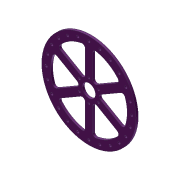
# Autodesk Inventor part: FlyWheelBase
Saved by Autodesk Inventor 2012 (Build 160160000, 160)
## iProperties
Created: 2012-01-20
Part Number: FlyWheelBase
Material: Aluminum-6061
Document SubType Name: Modeling
Designer: JesseK
Mass: 221.849 g
Surface Area: 457.511 cm^2
Volume: 81.8629 cm^3
Density: 2.71 g/cm^3
Author: JesseK
Autodesk Inventor part; units mm, degrees
ref_plane "YZ Plane" through (0, 0, 0) normal (1, 0, 0) x (0, 1, 0)
ref_plane "XZ Plane" through (0, 0, 0) normal (0, 1, 0) x (-1, 0, 0)
ref_plane "XY Plane" through (0, 0, 0) normal (0, 0, 1) x (1, 0, 0)
sketch "Sketch1" plane through (0, 0, 0) normal (0, 0, 1) x (1, 0, 0)
  circle A0 centre (0, 0) radius 101.6
  circle A1 centre (0, 0) radius 14.2875
  dimension "d0" = 203.2
  dimension "d1" = 28.575
  constraints: 2 centre point, 1 coincident
  measures "d0" diameter of A0
  measures "d1" diameter of A1
extrude "Extrusion1" add sketch "Sketch1" along normal blind 4.7625
sketch "Sketch4" plane through (0, 0, 4.7625) normal (0, 0, 1) x (1, 0, 0)
  circle A0 centre (0, 0) radius 101.6 projected
  circle A1 centre (0, 92.075) radius 2.8063
  line L0 (0, 0) -> (0, 101.6) construction
  circle A2 centre (0, 0) radius 92.075 construction
  dimension "d58" = 9.525
  constraints: 2 end point, 2 vertical alignment, 1 centre point, 1 coincident, 1 point on line, 1 vertical, 3 other
extrude "Extrusion5" cut sketch "Sketch4" against normal through all contours A1
pattern_circular "Circular Pattern3" count 24 over 360 about axis through (0, 0, -10) along (0, 0, 1) of "Extrusion5"
sketch "Sketch6" plane through (0, 0, 4.7625) normal (0, 0, 1) x (1, 0, 0)
  circle A0 centre (0, 0) radius 101.6 projected
  circle A1 centre (0, 23.8125) radius 2.3813
  circle A2 centre (0, 0) radius 23.8125 construction
  line L0 (0, 23.8125) -> (0, 0) construction
  dimension "d68" = 47.625
  dimension "d69" = 4.7625
  constraints: 2 end point, 1 centre point, 1 coincident, 1 vertical, 1 vertical alignment, 2 other
  measures "d69" diameter of A1
extrude "Extrusion6" cut sketch "Sketch6" against normal through all contours A1
pattern_circular "Circular Pattern4" count 6 over 360 about axis through (0, 0, -10) along (0, 0, 1) of "Extrusion6"
sketch "Sketch7" plane through (0, 0, 4.7625) normal (0, 0, 1) x (1, 0, 0)
  circle A0 centre (-20.6222, -11.9062) radius 2.3813 projected
  circle A1 centre (-20.6222, 11.9062) radius 2.3813 projected
  circle A2 centre (0, 23.8125) radius 2.3813 projected
  circle A3 centre (0, 0) radius 101.6 projected
  line L0 (0, 0) -> (0, 23.8125) construction
  line L1 (0, 23.8125) -> (0, 0) construction
  line L2 (-20.6222, 11.9062) -> (0, 0) construction
  line L3 (-20.6222, -11.9062) -> (0, 0) construction
  line L4 (-25.4, 5.4993) -> (-68.7895, 30.5502)
  line L5 (-68.7895, -30.5502) -> (-25.4, -5.4993)
  arc A4 (-77.9615, 27.1385) -> (-77.9615, -27.1385) centre (0, 0) ccw
  arc A5 (-68.7895, 30.5502) -> (-77.9615, 27.1385) centre (-71.9645, 25.0509) ccw
  arc A6 (-77.9615, -27.1385) -> (-68.7895, -30.5502) centre (-71.9645, -25.0509) ccw
  arc A7 (-25.4, -5.4993) -> (-25.4, 5.4993) centre (-28.575, 0) ccw
  point P0 (-75.1279, -34.2097)
  point P1 (-75.1279, 34.2097)
  dimension "d75" = 19.05
  dimension "d76" = 6.35
  dimension "d78" = 7.9375
  constraints: 12 end point, 10 point on circle, 6 tangent, 4 centre point, 2 equal radius, 2 parallel, 2 point on line, 2 vertical, 1 coincident, 1 equal length
  measures "d75" radial gap between concentric circles of A3 A4
  measures "d76" radius of A5
  measures "d78" distance between parallel lines of L2 L4
extrude "Extrusion7" cut sketch "Sketch7" against normal through all contours A7 L5 A6 A4 A5 L4
pattern_circular "Circular Pattern5" count 6 over 360 about axis through (0, 0, -10) along (0, 0, 1) of "Extrusion7"
body "Solid1"
